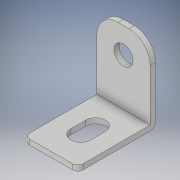
# Autodesk Inventor part: angle bracket short
Saved by Autodesk Inventor 2018 (Build 220112000, 112)
## iProperties
Created: 2018-06-25
Part Number: angle bracket short
Material: Generic
Document SubType Name: Modeling
Designer: Ajith Thomas
Density: 1 g/cm^3
Appearance: Default
Author: Ajith Thomas
Autodesk Inventor part; units mm, degrees
ref_plane "YZ Plane" through (0, 0, 0) normal (1, 0, 0) x (0, 1, 0)
ref_plane "XZ Plane" through (0, 0, 0) normal (0, 1, 0) x (-1, 0, 0)
ref_plane "XY Plane" through (0, 0, 0) normal (0, 0, 1) x (1, 0, 0)
sketch "Sketch1" plane through (0, 0, 0) normal (0, 1, 0) x (-1, 0, 0)
  line L0 (5, 7.3) -> (-5, 7.3)
  line L1 (-5, 7.3) -> (-5, -7.3)
  line L2 (-5, -7.3) -> (5, -7.3)
  line L3 (5, -7.3) -> (5, 7.3)
  line L4 (5, 7.3) -> (-5, -7.3) construction
  line L5 (-5, 7.3) -> (5, -7.3) construction
  point P0 (0, 0)
  dimension "d0" = 10
  dimension "d1" = 14.6
  constraints: 12 end point, 2 midpoint, 2 parallel, 1 horizontal, 1 perpendicular
  measures "d0" distance of L2.end L1.end
  measures "d1" distance of L1.end L0.end
extrude "Extrusion1" add sketch "Sketch1" along normal blind 1
sketch "Sketch2" plane through (5, 0, -7.3) normal (0, 0, -1) x (-1, 0, 0)
  line L0 (0, 0) -> (10, 0) projected
  line L1 (0, 0) -> (0, 14.7)
  line L2 (0, 14.7) -> (10, 14.7)
  line L3 (10, 14.7) -> (10, 0)
  point P0 (5, 0)
  dimension "d4" = 14.7
  constraints: 6 end point, 2 perpendicular, 1 vertical
  measures "d4" distance of L0.start L1.end
extrude "Extrusion2" add sketch "Sketch2" against normal blind 1
fillet "Fillet1" radius 4 2 edges at (5, 14.7, -6.8) (-5, 14.7, -6.8)
fillet "Fillet2" radius 1 2 edges at (-5, 0.5, 7.3) (5, 0.5, 7.3)
fillet "Fillet3" radius 1 1 edges at (0, 0, -7.3)
sketch "Sketch3" plane through (1, 14.7, -7.3) normal (0, 0, -1) x (-1, 0, 0)
  circle A0 centre (1, -4.8) radius 1.8
  line L0 (-4, -13.7) -> (-4, -4) projected
  line L1 (1, -3) -> (2.7418, -3) construction
  line L2 (2, 0) -> (0, 0) construction
  point P0 (1, -14.7)
  dimension "d12" = 3.6
  dimension "d10" = 5
  dimension "d11" = 3
  constraints: 2 end point, 2 horizontal, 1 vertical alignment, 2 other
  measures "d10" distance from line of L0 point (1, -4.8)
  measures "d11" distance between parallel lines of L2 L1
extrude "Extrusion3" cut sketch "Sketch3" against normal blind 1
sketch "Sketch4" plane through (0, 0, 0) normal (0, -1, 0) x (1, 0, 0)
  line L0 (5, 6.3) -> (5, -6.3) projected
  line L1 (0, 3.6) -> (1.5693, 3.6) construction
  line L2 (-4, 7.3) -> (4, 7.3) projected
  line L3 (0, -2.9) -> (1.85, -2.9) construction
  line L4 (1.85, 1.75) -> (1.85, -1.05)
  line L5 (-1.85, 1.75) -> (-1.85, -1.05)
  arc A0 (1.85, 1.75) -> (-1.85, 1.75) centre (0, 1.75) ccw
  arc A1 (-1.85, -1.05) -> (1.85, -1.05) centre (0, -1.05) ccw
  line L6 (-5, -6.3) -> (-5, 6.3) projected
  point P0 (0, 0)
  dimension "d16" = 5
  dimension "d17" = 3.7
  dimension "d19" = 6.5
  dimension "d20" = 3.15
  dimension "d21" = 3.15
  constraints: 8 end point, 6 point on circle, 5 tangent, 2 centre point, 2 horizontal, 2 vertical
  measures "d16" distance from line of L0 A0.centre
  measures "d17" distance between parallel lines of L2 L1
  measures "d19" distance between parallel lines of L1 L3
  measures "d20" distance between parallel lines of L6 L5
  measures "d21" distance between parallel lines of L0 L4
extrude "Extrusion4" cut sketch "Sketch4" against normal blind 1
body "Solid1"
